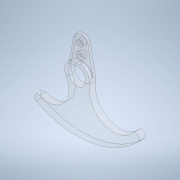
# Autodesk Inventor part: ヘッケン
Saved by Autodesk Inventor 2022.2 (Build 262287000, 287)
## iProperties
Created: 2022-01-09
Part Number: ヘッケン
Material: Polycarbonate, Clear
Document SubType Name: Modeling
Designer: acps
Density: 1.2 g/cm^3
Appearance: Polycarbonate - Clear
Author: acps
Autodesk Inventor part; units mm, degrees
ref_plane "YZ Plane" through (0, 0, 0) normal (1, 0, 0) x (0, 1, 0)
ref_plane "XZ Plane" through (0, 0, 0) normal (0, 1, 0) x (-1, 0, 0)
ref_plane "XY Plane" through (0, 0, 0) normal (0, 0, 1) x (1, 0, 0)
sketch "Sketch1" plane through (0, 0, 0) normal (0, 0, 1) x (1, 0, 0)
  line L0 (64.2929, 13) -> (99.1548, 4.0199) construction
  circle A0 centre (64.2929, 13) radius 3 construction
  circle A1 centre (64.2929, 13) radius 4.025 construction
  circle A2 centre (64.2929, 13) radius 7 construction
  arc A3 (102.6474, 8.8986) -> (63.8399, 19.9853) centre (67.7221, -39.8889) ccw construction
  circle A4 centre (99.1548, 4.0199) radius 2.5
  circle A5 centre (99.1548, 4.0199) radius 3.525
  circle A6 centre (99.1548, 4.0199) radius 6
  line L1 (64.2929, 13) -> (98.9408, 0.0186) construction
  line L2 (99.1548, 4.0199) -> (99.1548, -17.9801) construction
  line L3 (99.1548, -17.9801) -> (98.9408, 0.0186) construction
  circle A7 centre (99.1548, -17.9801) radius 10
  circle A8 centre (99.1548, -17.9801) radius 7.025
  line L4 (105.0548, 5.1108) -> (108.9881, -16.162)
  line L5 (93.2548, 5.1108) -> (89.3215, -16.162)
  line L6 (9.3628, -60) -> (214.5663, -60) construction
  arc A9 (95.4028, -0.6623) -> (65.8301, 6.1709) centre (73.5161, -27.9748) ccw construction
  line L7 (99.1548, 4.0199) -> (66.0447, -51.9827) construction
  line L8 (99.1548, 4.0199) -> (148.8226, -39.0251) construction
  circle A10 centre (67.5736, -49.3967) radius 3
  circle A11 centre (146.5507, -37.0561) radius 3
  arc A12 (68.7666, -46.6441) -> (90.4037, -22.8193) centre (75.5268, -31.046) ccw
  arc A13 (109.0459, -19.4522) -> (144.239, -35.1439) centre (128.828, -22.3964) ccw
  arc A14 (66.0447, -51.9827) -> (148.8226, -39.0251) centre (98.68, 10.4177) ccw
  circle A15 centre (99.1548, -4.9801) radius 1.25
  circle A16 centre (99.1548, -4.9801) radius 3
  circle A17 centre (99.1548, -4.9801) radius 4.25
  circle A18 centre (99.1548, 4.0199) radius 1.25
  point P0 (0, 0)
  point P1 (0, 0)
  point P2 (66.1895, -52.0583)
  point P3 (148.6808, -39.1685)
  point P4 (99.1548, -7.9801)
  point P5 (101.772, -8.3287)
  point P6 (96.5376, -8.3287)
  dimension "d19" = 6
  dimension "d20" = 6
  dimension "d0" = 36
  dimension "d1" = 8.05
  dimension "d2" = 6
  dimension "d3" = 14
  dimension "d4" = 60
  dimension "d5" = 37
  dimension "d6" = 22
  dimension "d7" = 18
  dimension "d8" = 12
  dimension "d9" = 7.05
  dimension "d10" = 20
  dimension "d11" = 14.05
  dimension "d12" = 35
  dimension "d13" = 5
  dimension "d14" = 60
  dimension "d15" = 30.593
  dimension "d16" = 49.086
  dimension "d17" = 65.7249
  dimension "d18" = 65.0582
  dimension "d21" = 13
  dimension "d22" = 70.4193
  dimension "d23" = 17
  dimension "d24" = 20
  dimension "d29" = 2.5
  dimension "d30" = 6
  dimension "d31" = 8.5
  dimension "d32" = 2.5
  constraints: 20 point on circle, 17 centre point, 16 end point, 11 coincident, 11 tangent, 3 point on line, 1 horizontal, 1 vertical, 15 other
  measures "d0" distance of L0.start L0.end
  measures "d1" diameter of A1
  measures "d2" diameter of A0
  measures "d3" diameter of A2
  measures "d4" radius of A3
  measures "d5" distance of L3.end A1.centre
  measures "d6" distance of L2.start L2.end
  measures "d7" distance of L3.end L2.end
  measures "d8" diameter of A6
  measures "d9" diameter of A5
  measures "d10" diameter of A7
  measures "d11" diameter of A8
  measures "d12" radius of A9
  measures "d13" diameter of A4
  measures "d14" distance from line of L6 point (0, 0)
  measures "d15" angle of L2 L7
  measures "d16" angle of L2 L8
  measures "d17" distance of L2.start L8.end
  measures "d18" distance of L2.start L7.end
  measures "d21" vertical distance of point (0, 0) L0.start
  measures "d22" radius of A14
  measures "d23" radius of A12
  measures "d24" radius of A13
  measures "d29" diameter of A15
  measures "d30" diameter of A16
  measures "d31" diameter of A17
  measures "d32" diameter of A18
extrude "Extrusion1" add sketch "Sketch1" along normal blind 5 contours A7 A17 | A7 A13 A11 A14 A10 A12 | A10 | A11 picked at (92.0551, -23.4279)
extrude "Extrusion3" add sketch "Sketch1" along normal blind 3 contours A4 | A16
extrude "Extrusion4" add sketch "Sketch1" along normal blind 2 contours A5 | A6 A17 | A6 L4 A7 A17 | A17 A7 A16 A6 | A6 A17 | A6 A17 A7 L5 | A16 A7 A17 A6 | A17 A7 picked at (98.8441, -8.7789)
chamfer "Chamfer1" distance 1.6 angle 45 1 edges at (97.9048, -4.9801, 0)
chamfer "Chamfer2" distance 1.6 angle 45 1 edges at (97.9048, 4.0199, 0)
body "Solid1"
